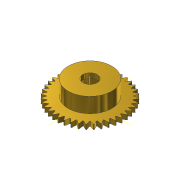
# Autodesk Inventor part: empty
Saved by Autodesk Inventor 2014 (Build 180170000, 170)
## iProperties
Created: 2015-04-13
Part Number: empty
Material: Generic
Document SubType Name: Modeling
Designer: Martin
Density: 1 g/cm^3
Appearance: Default
Author: Martin
Autodesk Inventor part; units mm, degrees
ref_plane "YZ Plane" through (0, 0, 0) normal (1, 0, 0) x (0, 1, 0)
ref_plane "XZ Plane" through (0, 0, 0) normal (0, 1, 0) x (-1, 0, 0)
ref_plane "XY Plane" through (0, 0, 0) normal (0, 0, 1) x (1, 0, 0)
sketch "Sketch1" plane through (0, 0, 0) normal (1, 0, 0) x (0, 1, 0)
  line L0 (0, -21.2618) -> (0, 40.0382) projected
  line L1 (-1.55, 0) -> (9.3, 0) projected
  line L2 (0, 31.281) -> (0, -12.5047)
  line L3 (1.6, 4.4) -> (1.6, 3.3)
  line L4 (1.6, 3.3) -> (3.95, 3.3)
  line L5 (3.95, 3.3) -> (3.95, 0)
  line L6 (3.95, 0) -> (7.75, 0)
  line L7 (7.75, 0) -> (7.75, 1.05)
  line L8 (7.75, 1.05) -> (4.85, 1.05)
  line L9 (4.85, 1.05) -> (4.85, 4.4)
  line L10 (4.85, 4.4) -> (1.6, 4.4)
  point P0 (0, 0)
  dimension "d0" = 1.05
  dimension "d1" = 4.4
  dimension "d2" = 9.7
  dimension "d3" = 7.9
  dimension "d4" = 3.3
  dimension "d5" = 3.2
  dimension "d16" = 15.5
  constraints: 18 end point, 4 perpendicular, 4 point on line, 3 parallel
  measures "d0" distance of L6.end L7.end
  measures "d1" distance between parallel lines of L1 L10
  measures "d2" diameter of L9 L2
  measures "d3" diameter of L5 L2
  measures "d4" distance between parallel lines of L1 L4
  measures "d5" diameter of L3 L2
  measures "d16" diameter of L7 L2
revolve "Revolution1" add sketch "Sketch1" angle 360 about axis through (0, 0, 31.281) along (0, 0, -1)
sketch "Sketch2" plane through (0, 0, 1.05) normal (0, 0, 1) x (1, 0, 0)
  circle A0 centre (0, 0) radius 7.75 projected
  line L0 (0, -14.3541) -> (0, 14.3541) projected
  line L1 (0, 0) -> (-0.6081, 7.7261) construction
  line L2 (0, 0) -> (0.6081, 7.7261) construction
  line L3 (-0.5426, 7.731) -> (0, 6.7123) construction
  line L4 (0, 6.7123) -> (0.5426, 7.731) construction
  arc A1 (-0.0883, 6.878) -> (0.0883, 6.878) centre (0, 6.925) ccw
  arc A2 (-0.512, 7.6734) -> (-0.6081, 7.7261) centre (-0.6002, 7.6264) ccw
  arc A3 (0.6081, 7.7261) -> (0.512, 7.6734) centre (0.6002, 7.6264) ccw
  line L5 (0, 6.925) -> (0, 7.75)
  line L6 (-0.512, 7.6734) -> (-0.0883, 6.878)
  line L7 (0.0883, 6.878) -> (0.512, 7.6734)
  dimension "d7" = 9
  dimension "d8" = 0.1
  dimension "d9" = 0.1
  dimension "d10" = 0.825
  constraints: 14 end point, 12 point on circle, 8 tangent, 7 point on line, 3 centre point, 2 collinear, 2 line through centre, 2 other
  measures "d7" angle of L2 L1
  measures "d8" radius of A2
  measures "d9" radius of A1
  measures "d10" distance of L5.start L5.end
extrude "Extrusion1" cut sketch "Sketch2" against normal through all contours A3 L7 A1 L0 A0 | L0 A1 L6 A2 A0 picked at (0.2677, 7.4329) picked at (-0.2677, 7.4329)
pattern_circular "Circular Pattern1" count 40 over 360 about axis through (0, 0, -10) along (0, 0, 1) of "Extrusion1"
body "Solid1"
